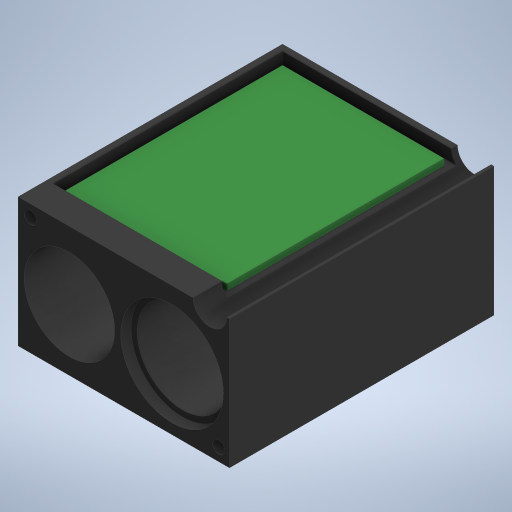
# Autodesk Inventor part: Small LRF Real
Saved by Autodesk Inventor 2024.1 (Build 281209000, 209)
## iProperties
Created: 2025-04-08
Part Number: Small LRF Real
Material: Generic
Document SubType Name: Modeling
Designer: User
Density: 1 g/cm^3
Appearance: Default
Author: User
Autodesk Inventor part; units mm, degrees
ref_plane "YZ Plane" through (0, 0, 0) normal (1, 0, 0) x (0, 1, 0)
ref_plane "XZ Plane" through (0, 0, 0) normal (0, 1, 0) x (-1, 0, 0)
ref_plane "XY Plane" through (0, 0, 0) normal (0, 0, 1) x (1, 0, 0)
sketch "Sketch1" plane through (0, 0, 0) normal (0, 1, 0) x (-1, 0, 0)
  line L0 (0, 0) -> (35, 0)
  line L1 (35, 0) -> (35, -43.79)
  line L2 (35, -43.79) -> (0, -43.79)
  line L3 (0, -43.79) -> (0, 0)
  dimension "d0" = 35
  dimension "d1" = 43.79
  constraints: 8 end point, 2 parallel, 1 horizontal, 1 perpendicular
  measures "d0" distance of L1.end L2.end
  measures "d1" distance of L0.end L1.end
extrude "Extrusion1" add sketch "Sketch1" along normal blind 21.37
sketch "Sketch2" plane through (-35, 0, 0) normal (0, 0, 1) x (1, 0, 0)
  circle A0 centre (8.49, 10.185) radius 7.5
  circle A1 centre (25.49, 10.185) radius 7.5
  point P0 (35, 0)
  dimension "d4" = 15
  dimension "d5" = 15
  constraints: 2 centre point
  measures "d4" diameter of A0
  measures "d5" diameter of A1
extrude "Extrusion2" cut sketch "Sketch2" against normal blind 35.79
sketch "Sketch3" plane through (-35, 0, 0) normal (0, 0, 1) x (1, 0, 0)
  circle A0 centre (25.49, 10.185) radius 7.5 projected
  circle A1 centre (25.49, 10.185) radius 8.5
  point P0 (35, 0)
  dimension "d9" = 17
  constraints: 1 centre point, 1 coincident
  measures "d9" diameter of A1
extrude "Extrusion3" cut sketch "Sketch3" against normal blind 1.73
sketch "Sketch4" plane through (-35, 0, 0) normal (0, 0, 1) x (1, 0, 0)
  circle A0 centre (2.02, 19.35) radius 1.02
  circle A1 centre (33.17, 2.02) radius 1.02
  point P0 (35, 0)
  dimension "d12" = 2.04
  dimension "d13" = 2.04
  constraints: 2 centre point
  measures "d12" diameter of A0
  measures "d13" diameter of A1
extrude "Extrusion4" cut sketch "Sketch4" against normal blind 2.1
sketch "Sketch5" plane through (0, 0, 0) normal (0, -1, 0) x (1, 0, 0)
  circle A0 centre (-32.19, -3) radius 1.02
  circle A1 centre (-3, -40.79) radius 1.02
  point P0 (0, 0)
  dimension "d17" = 2.04
  dimension "d23" = 2.04
  constraints: 2 centre point
  measures "d17" diameter of A0
  measures "d23" diameter of A1
extrude "Extrusion5" cut sketch "Sketch5" against normal blind 2.1
sketch "Sketch6" plane through (0, 0, 0) normal (0, -1, 0) x (1, 0, 0)
  circle A0 centre (-18.19, -15.39) radius 1.02
  circle A1 centre (-18.19, -31.79) radius 1.02
  point P0 (0, 0)
  dimension "d20" = 2.04
  dimension "d21" = 2.04
  constraints: 2 centre point
  measures "d20" diameter of A0
  measures "d21" diameter of A1
extrude "Extrusion6" cut sketch "Sketch6" against normal blind 6.1
sketch "Sketch10" plane through (0, 21.37, 0) normal (0, 1, 0) x (1, 0, 0)
  line L0 (-35, 43.79) -> (-35, 0) projected
  line L1 (0, 0) -> (0, 43.79) projected
  line L2 (-35, 43.79) -> (0, 43.79)
  line L3 (0, 43.79) -> (0, 3.79)
  line L4 (0, 3.79) -> (-35, 3.79)
  line L5 (-35, 3.79) -> (-35, 43.79)
  line L6 (-34, 4.79) -> (-1, 4.79)
  line L7 (-1, 4.79) -> (-1, 42.79)
  line L8 (-1, 42.79) -> (-34, 42.79)
  line L9 (-34, 42.79) -> (-34, 4.79)
  dimension "d30" = 40
  dimension "d31" = 1
  constraints: 16 end point, 4 parallel, 2 perpendicular, 1 horizontal, 1 point on line, 3 other
  measures "d30" distance of L2.end L3.end
  measures "d31" distance between parallel lines of L4 L6
extrude "Extrusion8" cut sketch "Sketch10" against normal blind 2 contours L9 L8 L7 L6
sketch "Sketch11" plane through (-35, 0, 0) normal (0, 0, 1) x (1, 0, 0)
  line L0 (35, 21.37) -> (0, 21.37) projected
  circle A0 centre (31.7551, 21.37) radius 2.79
  point P0 (35, 0)
  dimension "d34" = 5.58
  constraints: 1 centre point, 1 point on line
  measures "d34" diameter of A0
extrude "Extrusion9" cut sketch "Sketch11" against normal through all
sketch "Sketch12" plane through (0, 19.37, 0) normal (0, 1, 0) x (1, 0, 0)
  line L0 (-34, 4.79) -> (-34, 42.79) projected
  line L1 (-5.1902, 4.79) -> (-5.1902, 42.79) projected
  line L2 (-34, 42.79) -> (-5.1902, 42.79)
  line L3 (-5.1902, 42.79) -> (-5.1902, 4.79)
  line L4 (-5.1902, 4.79) -> (-34, 4.79)
  line L5 (-34, 4.79) -> (-34, 42.79)
  line L6 (-33, 5.79) -> (-6.1902, 5.79)
  line L7 (-6.1902, 5.79) -> (-6.1902, 41.79)
  line L8 (-6.1902, 41.79) -> (-33, 41.79)
  line L9 (-33, 41.79) -> (-33, 5.79)
  point P0 (0, 0)
  dimension "d37" = 1
  constraints: 16 end point, 4 parallel, 2 perpendicular, 1 horizontal, 3 other
  measures "d37" distance between parallel lines of L4 L6
extrude "Extrusion10" add sketch "Sketch12" along normal blind 1 contours L9 L8 L7 L6
body "Solid1"
